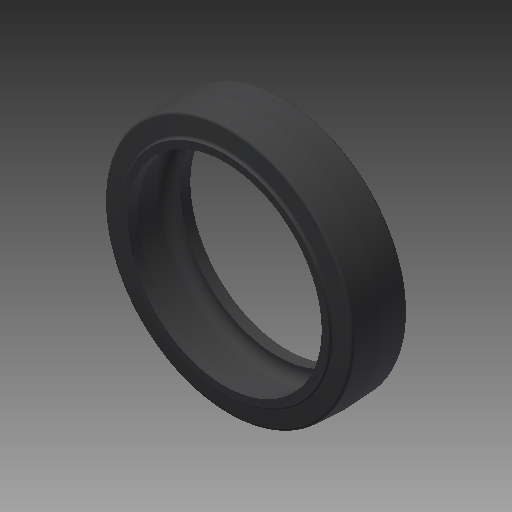
# Autodesk Inventor part: 3.00006.4411 1/2 (T)
Saved by Autodesk Inventor 2018 (Build 220112000, 112)
## iProperties
Category: PARTsolutions
Company: COLSONGROUP
Created: 2018-01-09
Part Number: 3.00006.4411 1/2 (T)
Catalog Web Link: www.cadenas.de
Description: Performa Rubber T-Wheels - Capacity up to 1700 lbs Each
Vendor: COLSONGROUP
Document SubType Name: Modeling
Designer: psAdmin
Manufacturer: COLSONGROUP
Mass: 177.567 g
Surface Area: 491.659 cm^2
Volume: 177.567 cm^3
Density: 1 g/cm^3
Material: Generic
Appearance: PSOLRGB-127-127-127
PSOL_IDENT_0: {$CADENAS_DATA\23d-libs\colsongroup\colson\wheels\performa_rubber\performa_rubber_thread.prj},209 {V
PSOL_IDENT_1: TYP=3D},{NB=3.00006.4411 1/2 (T)},{LINA=3.00006.4411 1/2 (T)},{NN=Performa Rubber T},{DATE=12.06.201
PSOL_IDENT_2: 7 06:51:29},{GEOMDATE=09.06.2017 06:04:53},{VERSION=},{LINEID=10},{LINESUBID=-1},{WBVAR=WT,SER,D,W,W
PSOL_IDENT_3: B,TG}  {NB=3.00006.4411 1/2 (T)},{LINA=3.00006.4411 1/2 (T)},{KT=DUMMY},{PN=3.00006.4411 1/2},{WH=Pe
PSOL_IDENT_4: rforma Rubber},{WT=PRFG},{SER=3},{SERALG= '1','1 Series (Capacity up to 145 lbs)','2','2 Series (Cap
PSOL_IDENT_5: acity up to 325 lbs)','3','3 Series (Capacity up to 375 lbs)','4','4 Series (Capacity up to 500 lbs)'
PSOL_IDENT_6: ,'5','5 Series (Capacity up to 675 lbs)' },{D=6.00000000},{DALG=3,4,5,6},{DPN=06},{W=1.50000000},{WA
PSOL_IDENT_7: LG=1.5},{WTPN1=4},{WTPN2=4},{WTPN3=},{CAP=375},{CAPALG=375},{CAPPN=},{WB=1},{WBALG= '1','Delrin','9'
PSOL_IDENT_8: ,'Roller','5','PPBB' },{WBPN=441},{TG=-},{TGALG= '-','N/A' },{TGPN=},{BB=0.50000000},{LBB=1.18750000
PSOL_IDENT_9: },{HUB=1.62500000},{SBB=0.37500000},{SBL=1.87500000},{WEIGHT=1.50000000},{CON=3},{D1=1.63},{D2=4.64}
PSOL_IDENT_10: ,{BORE=1.19},{ANGS=5},{ANGT=3},{R1=0.25},{TT=0.31},{W1=0.25},{D3=3.93},{T=0.56},{ANGD=5},{ANGU=5},{T
PSOL_IDENT_11: 2=0.19},{T3=0.17},{R2=0.0625},{W2=1.25},{COLOR=0.50,0.50,0.50,0.00},{TT1=0.31}
NN: Performa Rubber T
NT: Wheels - Capacity up to 1700 lbs Each
NB: 3.00006.4411 1/2 (T)
NBSYN: $PN. (T)
LINA: 3.00006.4411 1/2 (T)
PN: 3.00006.4411 1/2
WH: Performa Rubber
WT: Flat Gray Thread
SER: 3 Series (Capacity up to 375 lbs)
D: 6
W: 1 1/2
WB: Delrin
TG: N/A
BB: 1/2
LBB: 1 3/16
HUB: 1 5/8
SBB: 3/8
SBL: 1 7/8
WEIGHT: 1 1/2
SUPPLIER: COLSONGROUP
ARTICLENO: 3.00006.4411 1/2 (T)
BOMINFO: 3.00006.4411 1/2 (T)
CREATOR: CADENAS GmbH
Title: 3.00006.4411 1/2 (T)
Author: Cadenas PARTsolutions
Comments: Wheels - Capacity up to 1700 lbs Each
Autodesk Inventor part; units mm, degrees
sketch "Sketch_8" plane through (0, 0, 0) normal (1, 0, 0) x (0, 1, 0)
  line L0 (0, -19.05) -> (0, 19.05)
  line L1 (58.928, 19.05) -> (58.928, 12.7)
  line L2 (58.928, 12.7) -> (60.452, 12.7)
  arc A0 (66.802, 6.35) -> (60.452, 12.7) centre (60.452, 6.35) ccw
  line L3 (66.802, 6.35) -> (66.802, -6.35)
  arc A1 (60.452, -12.7) -> (66.802, -6.35) centre (60.452, -6.35) ccw
  line L4 (60.452, -12.7) -> (58.928, -12.7)
  line L5 (58.928, -12.7) -> (58.928, -19.05)
  line L6 (58.928, -19.05) -> (63.246, -19.05)
  arc A2 (64.8335, -17.4625) -> (63.246, -19.05) centre (64.8335, -19.05) ccw
  line L7 (64.8335, -17.4625) -> (73.9582, -16.6642)
  arc A3 (73.9582, -16.6642) -> (75.4052, -15.1658) centre (73.8199, -15.0827) ccw
  line L8 (75.4052, -15.1658) -> (76.2, 0)
  line L9 (76.2, 0) -> (75.4052, 15.1658)
  arc A4 (75.4052, 15.1658) -> (73.9582, 16.6642) centre (73.8199, 15.0827) ccw
  line L10 (73.9582, 16.6642) -> (64.8335, 17.4625)
  arc A5 (63.246, 19.05) -> (64.8335, 17.4625) centre (64.8335, 19.05) ccw
  line L11 (63.246, 19.05) -> (58.928, 19.05)
  constraints: 24 end point, 12 point on circle, 6 centre point
revolve "Revolution1" add sketch "Sketch_8" angle 360 about axis through (0, 0, -19.05) along (0, 0, -1)
ref_plane "thread_XY" through (0, 0, 0) normal (0, 0, 1) x (1, 0, 0)
ref_plane "thread_YZ" through (0, 0, 0) normal (1, 0, 0) x (0, 1, 0)
ref_plane "thread_ZX" through (0, 0, 0) normal (0, 1, 0) x (0, 0, 1)
body "Solid1"
